Autodesk Fusion 360 part; units mm, degrees
(part 2 of 3)
sketch "plate_cut" plane through (0, 0, 0) normal (0, 1, 0) x (1, 0, 0)
  arc A0 (26.05, -31.55) -> (25.05, -32.55) centre (25.05, -31.55) cw
  arc A1 (13.05, -32.55) -> (12.05, -31.55) centre (13.05, -31.55) cw
  line L0 (1.286, -37.6) -> (13.286, -37.6)
  line L1 (14.286, -38.6) -> (14.286, -50.6)
  line L2 (23.2714, -39.7827) -> (20.1656, -51.3738)
  arc A2 (14.286, -50.6) -> (13.286, -51.6) centre (13.286, -50.6) cw
  arc A3 (36.7944, -43.4062) -> (36.0873, -42.1814) centre (35.8285, -43.1474) ccw
  arc A4 (32.4638, -55.7044) -> (33.6886, -54.9973) centre (32.7226, -54.7385) ccw
  arc A5 (13.286, -37.6) -> (14.286, -38.6) centre (13.286, -38.6) cw
  arc A6 (24.4962, -39.0756) -> (23.2714, -39.7827) centre (24.2374, -40.0415) ccw
  line L3 (59.2962, -48.3878) -> (48.9038, -42.3878)
  line L4 (25.05, -32.55) -> (13.05, -32.55)
  arc A7 (32.1, -35.05) -> (31.1, -34.05) centre (32.1, -34.05) cw
  arc A8 (20.1656, -51.3738) -> (20.8727, -52.5986) centre (21.1315, -51.6326) ccw
  line L5 (20.8727, -52.5986) -> (32.4638, -55.7044)
  line L6 (13.286, -51.6) -> (1.286, -51.6)
  arc A9 (-7, 6) -> (-6, 7) centre (-6, 6) cw
  line L7 (-13.05, 6.05) -> (-25.05, 6.05)
  line L8 (-7, -6) -> (-7, 6)
  line L9 (47.5378, -42.7538) -> (41.5378, -53.1462)
  arc A10 (26.05, -12.5) -> (25.05, -13.5) centre (25.05, -12.5) cw
  arc A11 (6, 7) -> (7, 6) centre (6, 6) cw
  line L10 (-12.05, -19.06) -> (-12.05, -31.06)
  arc A12 (12.05, -19.55) -> (13.05, -18.55) centre (13.05, -19.55) cw
  line L11 (45.1, -22.05) -> (45.1, -34.05)
  arc A13 (-12.05, 7.05) -> (-13.05, 6.05) centre (-13.05, 7.05) cw
  arc A14 (-6, -26.05) -> (-7, -25.05) centre (-6, -25.05) cw
  arc A15 (1.286, -51.6) -> (0.286, -50.6) centre (1.286, -50.6) cw
  arc A16 (-13.05, -18.06) -> (-12.05, -19.06) centre (-13.05, -19.06) cw
  arc A17 (-13.05, 1) -> (-12.05, 0) centre (-13.05, 0) cw
  line L12 (12.05, -12.5) -> (12.05, -0.5)
  line L13 (6, -26.05) -> (-6, -26.05)
  line L14 (-25.05, 1) -> (-13.05, 1)
  arc A18 (-6, -7) -> (-7, -6) centre (-6, -6) cw
  arc A19 (12.05, -0.5) -> (13.05, 0.5) centre (13.05, -0.5) cw
  line L15 (7, -13.05) -> (7, -25.05)
  line L16 (-45.1, -43.05) -> (-45.1, -31.05)
  line L17 (-32.1, -25) -> (-44.1, -25)
  line L18 (53.6622, -60.1462) -> (59.6622, -49.7538)
  arc A20 (41.5378, -53.1462) -> (41.9038, -54.5122) centre (42.4038, -53.6462) ccw
  line L19 (13.05, 0.5) -> (25.05, 0.5)
  arc A21 (-26.05, -19.06) -> (-25.05, -18.06) centre (-25.05, -19.06) cw
  line L20 (44.1, 3.05) -> (32.1, 3.05)
  line L21 (-44.1, -30.05) -> (-32.1, -30.05)
  arc A22 (-45.1, -12) -> (-44.1, -11) centre (-44.1, -12) cw
  arc A23 (13.05, 5.55) -> (12.05, 6.55) centre (13.05, 6.55) cw
  arc A24 (25.05, -18.55) -> (26.05, -19.55) centre (25.05, -19.55) cw
  line L22 (-6, 7) -> (6, 7)
  arc A25 (-32.1, -30.05) -> (-31.1, -31.05) centre (-32.1, -31.05) cw
  line L23 (31.1, 4.05) -> (31.1, 16.05)
  line L24 (-31.1, -31.05) -> (-31.1, -43.05)
  line L25 (32.1, 17.05) -> (44.1, 17.05)
  line L26 (12.05, 6.55) -> (12.05, 18.55)
  line L27 (26.05, 18.55) -> (26.05, 6.55)
  line L28 (-44.1, -11) -> (-32.1, -11)
  line L29 (25.05, 5.55) -> (13.05, 5.55)
  arc A26 (45.1, 4.05) -> (44.1, 3.05) centre (44.1, 4.05) cw
  line L30 (-32.1, -44.05) -> (-44.1, -44.05)
  arc A27 (32.1, 3.05) -> (31.1, 4.05) centre (32.1, 4.05) cw
  line L31 (13.05, 19.55) -> (25.05, 19.55)
  line L32 (45.1, 16.05) -> (45.1, 4.05)
  line L33 (41.9038, -54.5122) -> (52.2962, -60.5122)
  line L34 (-12.05, 0) -> (-12.05, -12)
  line L35 (-26.05, -12) -> (-26.05, 0)
  arc A28 (59.6622, -49.7538) -> (59.2962, -48.3878) centre (58.7962, -49.2538) ccw
  arc A29 (48.9038, -42.3878) -> (47.5378, -42.7538) centre (48.4038, -43.2538) ccw
  line L36 (44.1, -35.05) -> (32.1, -35.05)
  line L37 (36.0873, -42.1814) -> (24.4962, -39.0756)
  line L38 (33.6886, -54.9973) -> (36.7944, -43.4062)
  line L39 (-7, -25.05) -> (-7, -13.05)
  arc A30 (25.05, 0.5) -> (26.05, -0.5) centre (25.05, -0.5) cw
  arc A31 (44.1, 17.05) -> (45.1, 16.05) centre (44.1, 16.05) cw
  arc A32 (45.1, -34.05) -> (44.1, -35.05) centre (44.1, -34.05) cw
  arc A33 (0.286, -38.6) -> (1.286, -37.6) centre (1.286, -38.6) cw
  arc A34 (7, -6) -> (6, -7) centre (6, -6) cw
  line L40 (-25.05, 20.05) -> (-13.05, 20.05)
  line L41 (6, -7) -> (-6, -7)
  arc A35 (13.05, -13.5) -> (12.05, -12.5) centre (13.05, -12.5) cw
  arc A36 (7, -25.05) -> (6, -26.05) centre (6, -25.05) cw
  line L42 (13.05, -18.55) -> (25.05, -18.55)
  line L43 (7, 6) -> (7, -6)
  line L44 (25.05, -13.5) -> (13.05, -13.5)
  arc A37 (-7, -13.05) -> (-6, -12.05) centre (-6, -13.05) cw
  line L45 (26.05, -0.5) -> (26.05, -12.5)
  arc A38 (6, -12.05) -> (7, -13.05) centre (6, -13.05) cw
  arc A39 (-12.05, -12) -> (-13.05, -13) centre (-13.05, -12) cw
  line L46 (0.286, -50.6) -> (0.286, -38.6)
  arc A40 (-12.05, -31.06) -> (-13.05, -32.06) centre (-13.05, -31.06) cw
  line L47 (26.05, -19.55) -> (26.05, -31.55)
  line L48 (-6, -12.05) -> (6, -12.05)
  line L49 (-6, 26.05) -> (6, 26.05)
  arc A41 (32.1, -16) -> (31.1, -15) centre (32.1, -15) cw
  line L50 (32.1, -21.05) -> (44.1, -21.05)
  line L51 (7, 25.05) -> (7, 13.05)
  arc A42 (44.1, -21.05) -> (45.1, -22.05) centre (44.1, -22.05) cw
  arc A43 (-26.05, 19.05) -> (-25.05, 20.05) centre (-25.05, 19.05) cw
  arc A44 (7, 13.05) -> (6, 12.05) centre (6, 13.05) cw
  arc A45 (31.1, -22.05) -> (32.1, -21.05) centre (32.1, -22.05) cw
  arc A46 (-44.1, 8.05) -> (-45.1, 7.05) centre (-44.1, 7.05) ccw
  line L52 (44.1, -16) -> (32.1, -16)
  arc A47 (-25.05, 6.05) -> (-26.05, 7.05) centre (-25.05, 7.05) cw
  arc A48 (-13.05, 20.05) -> (-12.05, 19.05) centre (-13.05, 19.05) cw
  line L53 (32.1, -2) -> (44.1, -2)
  arc A49 (31.1, -3) -> (32.1, -2) centre (32.1, -3) cw
  line L54 (-26.05, 7.05) -> (-26.05, 19.05)
  line L55 (31.1, -15) -> (31.1, -3)
  arc A50 (45.1, -15) -> (44.1, -16) centre (44.1, -15) cw
  arc A51 (6, 26.05) -> (7, 25.05) centre (6, 25.05) cw
  line L56 (-31.1, -4.95) -> (-31.1, 7.05)
  line L57 (-31.1, -12) -> (-31.1, -24)
  arc A52 (44.1, -2) -> (45.1, -3) centre (44.1, -3) cw
  line L58 (-44.1, -5.95) -> (-32.1, -5.95)
  arc A53 (-32.1, -11) -> (-31.1, -12) centre (-32.1, -12) cw
  arc A54 (-32.1, -5.95) -> (-31.1, -4.95) centre (-32.1, -4.95) ccw
  line L59 (45.1, -3) -> (45.1, -15)
  line L60 (-7, 13.05) -> (-7, 25.05)
  arc A55 (-7, 25.05) -> (-6, 26.05) centre (-6, 25.05) cw
  arc A56 (-44.1, -25) -> (-45.1, -24) centre (-44.1, -24) cw
  line L61 (-26.05, -31.06) -> (-26.05, -19.06)
  arc A57 (-6, 12.05) -> (-7, 13.05) centre (-6, 13.05) cw
  line L62 (-45.1, 7.05) -> (-45.1, -4.95)
  arc A58 (-25.05, -32.06) -> (-26.05, -31.06) centre (-25.05, -31.06) cw
  line L63 (-32.1, 8.05) -> (-44.1, 8.05)
  line L64 (6, 12.05) -> (-6, 12.05)
  arc A59 (-31.1, -43.05) -> (-32.1, -44.05) centre (-32.1, -43.05) cw
  arc A60 (-26.05, 0) -> (-25.05, 1) centre (-25.05, 0) cw
  arc A61 (-31.1, -24) -> (-32.1, -25) centre (-32.1, -24) cw
  line L65 (-12.05, 19.05) -> (-12.05, 7.05)
  arc A62 (25.05, 19.55) -> (26.05, 18.55) centre (25.05, 18.55) cw
  arc A63 (12.05, 18.55) -> (13.05, 19.55) centre (13.05, 18.55) cw
  line L66 (-45.1, -24) -> (-45.1, -12)
  arc A64 (-31.1, 7.05) -> (-32.1, 8.05) centre (-32.1, 7.05) ccw
  line L67 (-25.05, -18.06) -> (-13.05, -18.06)
  arc A65 (31.1, 16.05) -> (32.1, 17.05) centre (32.1, 16.05) cw
  arc A66 (-45.1, -31.05) -> (-44.1, -30.05) centre (-44.1, -31.05) cw
  line L68 (31.1, -34.05) -> (31.1, -22.05)
  arc A67 (-45.1, -4.95) -> (-44.1, -5.95) centre (-44.1, -4.95) ccw
  line L69 (-13.05, -32.06) -> (-25.05, -32.06)
  arc A68 (26.05, 6.55) -> (25.05, 5.55) centre (25.05, 6.55) cw
  arc A69 (-25.05, -13) -> (-26.05, -12) centre (-25.05, -12) cw
  line L70 (-13.05, -13) -> (-25.05, -13)
  line L71 (12.05, -31.55) -> (12.05, -19.55)
  arc A70 (-44.1, -44.05) -> (-45.1, -43.05) centre (-44.1, -43.05) cw
  arc A71 (52.2962, -60.5122) -> (53.6622, -60.1462) centre (52.7962, -59.6462) ccw
  arc A72 (-55.7487, 17.9209) -> (-60.125, 9.652) centre (-50.125, 9.652) ccw
  line L72 (-55.7487, 17.9209) -> (-24.2468, 39.3454)
  arc A73 (-18.6222, 41.0765) -> (-24.2468, 39.3454) centre (-18.6231, 31.0765) ccw
  line L73 (-18.6222, 41.0765) -> (18.4843, 41.0734)
  arc A74 (20.6567, 40.8344) -> (18.4843, 41.0734) centre (18.4835, 31.0734) ccw
  arc A75 (81.043, 19.3715) -> (73.2162, 29.1325) centre (71.043, 19.3715) ccw
  arc A76 (79.7028, -45.0985) -> (81.043, -40.0977) centre (71.043, -40.0977) ccw
  line L74 (79.7028, -45.0985) -> (61.8222, -76.0618)
  arc A77 (53.2987, -81.06) -> (61.8222, -76.0618) centre (53.1625, -71.0609) ccw
  line L75 (53.2987, -81.06) -> (29.1948, -81.3885)
  arc A78 (24.8527, -80.462) -> (29.1948, -81.3885) centre (29.0585, -71.3894) ccw
  line L76 (24.8527, -80.462) -> (-19.2813, -60.0025)
  arc A79 (-19.2813, -60.0025) -> (-23.4871, -59.075) centre (-23.4871, -69.075) ccw
  line L77 (-50.125, -59.075) -> (-23.4871, -59.075)
  arc A80 (-60.125, -49.075) -> (-50.125, -59.075) centre (-50.125, -49.075) ccw
  line L78 (-60.125, -49.075) -> (-60.125, 9.652)
  line L79 (20.6567, 40.8344) -> (46.8423, 35.0044)
  line L80 (81.043, 19.3715) -> (81.043, -25.8559)
  arc A81 (47.625, 34.0283) -> (46.8423, 35.0044) centre (46.625, 34.0283) ccw
  line L81 (47.625, 34.0283) -> (47.625, -32.5721)
  line L82 (69.2205, -25.8646) -> (69.0694, 28.8059)
  arc A82 (70.2867, 29.7847) -> (69.0694, 28.8059) centre (70.0694, 28.8086) ccw
  arc A83 (47.625, -32.5721) -> (48.1249, -33.4381) centre (48.625, -32.5721) ccw
  line L83 (48.1249, -33.4381) -> (57.1204, -38.6328)
  arc A84 (57.1204, -38.6328) -> (57.6205, -38.7668) centre (57.6205, -37.7668) ccw
  line L84 (70.2211, -26.8618) -> (80.0436, -26.8559)
  arc A85 (69.2205, -25.8646) -> (70.2211, -26.8618) centre (70.2205, -25.8618) ccw
  arc A86 (80.0436, -26.8559) -> (81.043, -25.8559) centre (80.043, -25.8559) ccw
  line L85 (57.6205, -38.7668) -> (80.043, -38.7668)
  arc A87 (81.043, -39.7668) -> (80.043, -38.7668) centre (80.043, -39.7668) ccw
  line L86 (81.043, -39.7668) -> (81.043, -40.0977)
  circle A88 centre (71.1231, -41.9588) radius 1.7
  circle A89 centre (53.7342, -72.0705) radius 1.7
  circle A90 centre (28.4977, -72.2317) radius 1.7
  circle A91 centre (-18.212, -50.5781) radius 1.7
  circle A92 centre (-51.125, -50.075) radius 1.7
  circle A93 centre (-51.125, 10.1813) radius 1.7
  circle A94 centre (-18.9309, 32.0765) radius 1.7
  circle A95 centre (18.5935, 32.0734) radius 1.7
  circle A96 centre (43.1794, 26.5995) radius 1.7
  circle A97 centre (72.0934, 20.1391) radius 1.7
  circle A98 centre (72.2122, -22.8606) radius 1.7
  line L87 (70.2867, 29.7847) -> (73.2162, 29.1325)
sketch "curve_measure" plane through (0, 0, 0) normal (0, 0, 1) x (1, 0, 0)
  line L0 (75, 8.5) -> (75, -1.5)
  line L1 (75, -1.5) -> (81, -1.5)
  line L2 (81, -1.5) -> (81, 8.5)
  line L3 (81, 8.5) -> (75, 8.5)
  line L4 (73.5, 6) -> (82.5, 6) construction
  line L5 (82, 3) -> (73.5, 3) construction
  line L6 (79.7028, 0) -> (61.8222, 0) construction
  line L7 (80.5, -0.5199) -> (80.5, 9.6972) construction
  line L8 (79.25, 9.8527) -> (79.25, -0.7376) construction
  dimension "d106" = 3
  dimension "d107" = 2.5
  dimension "d108" = 0.5
  dimension "d109" = 1.75
  dimension "d110" = 6
  constraint vertical L0
  constraint perpendicular L0 L1
  constraint perpendicular L1 L2
  constraint perpendicular L0 L3
  constraint perpendicular L2 L4
  constraint perpendicular L0 L5
  constraint perpendicular L3 L7
  constraint vertical L8
  measures "d106" distance of L5 L6
  measures "d107" distance of L3 L4
  measures "d108" distance of L2 L7
  measures "d109" distance of L2 L8
  measures "d110" distance of L0 L2
extrude "Extrude2" add sketch "plate_cut" against normal blind 1.6 makes body 1 at (2.2858, 0, 64.0215) makes body 2 at (75.5302, 0, -5.55)
sketch "key_outline" plane through (0, 0, 0) normal (0, 1, 0) x (1, 0, 0)
  line L0 (-47.625, 10.575) -> (-28.575, 10.575)
  line L1 (-28.575, 10.575) -> (-28.575, 22.575)
  line L2 (-28.575, 22.575) -> (-9.525, 22.575)
  line L3 (-9.525, 22.575) -> (-9.525, 28.575)
  line L4 (-9.525, 28.575) -> (9.525, 28.575)
  line L5 (9.525, 28.575) -> (9.525, 22.075)
  line L6 (9.525, 22.075) -> (28.575, 22.075)
  line L7 (28.575, 22.075) -> (28.575, 19.575)
  line L8 (28.575, 19.575) -> (47.625, 19.575)
  line L9 (47.625, 19.575) -> (47.625, -33.2267)
  line L10 (47.625, -33.2267) -> (65.9971, -43.8338)
  line L11 (65.9971, -43.8338) -> (51.7096, -68.5805)
  line L12 (51.7096, -68.5805) -> (35.2118, -59.0555)
  line L13 (35.2118, -59.0555) -> (16.8109, -54.125)
  line L14 (16.8109, -54.125) -> (-2.2391, -54.125)
  line L15 (-2.2391, -54.125) -> (-2.2391, -35.075)
  line L16 (-9.525, -34.575) -> (-28.575, -34.575)
  line L17 (-28.575, -34.575) -> (-28.575, -46.575)
  line L18 (-28.575, -46.575) -> (-47.625, -46.575)
  line L19 (-47.625, -46.575) -> (-47.625, 10.575)
  line L20 (-2.2391, -35.075) -> (-2.2391, -34.575)
  line L21 (-9.525, -34.575) -> (-2.2391, -34.575)
  line L22 (-9.525, -35.575) -> (-3.2391, -35.575)
  line L23 (-9.525, -35.575) -> (-27.575, -35.575)
  line L24 (-27.575, -35.575) -> (-27.575, -47.575)
  line L25 (-27.575, -47.575) -> (-48.625, -47.575)
  line L26 (-48.625, -47.575) -> (-48.625, 11.575)
  line L27 (-48.625, 11.575) -> (-29.575, 11.575)
  line L28 (-29.575, 11.575) -> (-29.575, 23.575)
  line L29 (-29.575, 23.575) -> (-10.525, 23.575)
  line L30 (-10.525, 23.575) -> (-10.525, 29.575)
  line L31 (-10.525, 29.575) -> (10.525, 29.575)
  line L32 (10.525, 29.575) -> (10.525, 23.075)
  line L33 (10.525, 23.075) -> (29.575, 23.075)
  line L34 (29.575, 23.075) -> (29.575, 20.575)
  line L35 (29.575, 20.575) -> (48.625, 20.575)
  line L36 (48.625, 20.575) -> (48.625, -32.6494)
  line L37 (48.625, -32.6494) -> (67.3631, -43.4678)
  line L38 (67.3631, -43.4678) -> (52.0756, -69.9465)
  line L39 (52.0756, -69.9465) -> (34.8258, -59.9874)
  line L40 (34.8258, -59.9874) -> (16.6792, -55.125)
  line L41 (16.6792, -55.125) -> (-3.2391, -55.125)
  line L42 (-3.2391, -55.125) -> (-3.2391, -35.575)
  point P0 (-47.625, 10.575)
  point P1 (-28.575, 10.575)
  point P2 (-28.575, 22.575)
  point P3 (-9.525, 22.575)
  point P4 (-9.525, 28.575)
  point P5 (9.525, 28.575)
  point P6 (9.525, 22.075)
  point P7 (28.575, 22.075)
  point P8 (28.575, 19.575)
  point P9 (47.625, 19.575)
  point P10 (47.625, -33.2267)
  point P11 (65.9971, -43.8338)
  point P12 (51.7096, -68.5805)
  point P13 (35.2118, -59.0555)
  point P14 (16.8109, -54.125)
  point P15 (-2.2391, -54.125)
  point P16 (-2.2391, -35.075)
  point P17 (-9.525, -34.575)
  point P18 (-28.575, -34.575)
  point P19 (-28.575, -46.575)
  point P20 (-47.625, -46.575)
  dimension "d128" = 1
  constraint coincident P0 L0.start
  constraint coincident P1 L0.end
  constraint coincident P2 L1.end
  constraint coincident P3 L2.end
  constraint coincident P4 L3.end
  constraint coincident P5 L4.end
  constraint coincident P6 L5.end
  constraint coincident P7 L6.end
  constraint coincident P8 L7.end
  constraint coincident P9 L8.end
  constraint coincident P10 L9.end
  constraint coincident P11 L10.end
  constraint coincident P12 L11.end
  constraint coincident P13 L12.end
  constraint coincident P14 L13.end
  constraint coincident P15 L14.end
  constraint coincident P16 L15.end
  constraint coincident P17 L16.start
  constraint coincident P18 L16.end
  constraint coincident P19 L17.end
  constraint coincident P20 L18.end
sketch "top_c" plane through (0, 0, 0) normal (0, 1, 0) x (1, 0, 0)
  line L0 (-48.625, 11.575) -> (-29.575, 11.575)
  line L1 (-48.625, -47.575) -> (-48.625, 11.575)
  line L2 (-29.575, 11.575) -> (-29.575, 23.575)
  line L3 (-29.575, 23.575) -> (-10.525, 23.575)
  line L4 (-10.525, 29.575) -> (10.525, 29.575)
  line L5 (-10.525, 23.575) -> (-10.525, 29.575)
  line L6 (10.525, 29.575) -> (10.525, 23.075)
  line L7 (10.525, 23.075) -> (29.575, 23.075)
  line L8 (29.575, 23.075) -> (29.575, 20.575)
  line L9 (29.575, 20.575) -> (48.625, 20.575)
  line L10 (48.625, 20.575) -> (48.625, -32.6494)
  line L11 (48.625, -32.6494) -> (67.3631, -43.4678)
  line L12 (67.3631, -43.4678) -> (52.0756, -69.9465)
  line L13 (52.0756, -69.9465) -> (34.8258, -59.9874)
  line L14 (34.8258, -59.9874) -> (16.6792, -55.125)
  line L15 (16.6792, -55.125) -> (-3.2391, -55.125)
  line L16 (-3.2391, -55.125) -> (-3.2391, -35.575)
  line L17 (-9.525, -35.575) -> (-3.2391, -35.575)
  line L18 (-9.525, -35.575) -> (-27.575, -35.575)
  line L19 (-27.575, -35.575) -> (-27.575, -47.575)
  line L20 (-27.575, -47.575) -> (-48.625, -47.575)
  line L21 (-18.6227, 35.5765) -> (18.4839, 35.5734)
  arc A0 (19.4614, 35.4658) -> (18.4839, 35.5734) centre (18.4835, 31.0734) ccw
  line L22 (19.4614, 35.4658) -> (45.6471, 29.6358)
  circle A1 centre (18.5935, 32.0734) radius 1.1
  circle A2 centre (43.1794, 26.5995) radius 1.1
  circle A3 centre (-18.9309, 32.0765) radius 1.1
  arc A4 (-18.6227, 35.5765) -> (-21.1537, 34.7975) centre (-18.6231, 31.0765) ccw
  line L23 (-52.6557, 13.373) -> (-21.1537, 34.7975)
  line L24 (45.6471, 29.6358) -> (70.2803, 24.3774)
  line L25 (72.0209, 23.7639) -> (70.2803, 24.3774)
  arc A5 (75.543, 19.3715) -> (72.0209, 23.7639) centre (71.043, 19.3715) ccw
  circle A6 centre (72.0934, 20.1391) radius 1.1
  line L26 (75.543, 19.3715) -> (75.543, -25.8607)
  line L27 (75.543, -25.8607) -> (75.543, -40.0977)
  arc A7 (74.9399, -42.3481) -> (75.543, -40.0977) centre (71.043, -40.0977) ccw
  line L28 (74.9399, -42.3481) -> (57.0594, -73.3113)
  arc A8 (53.2238, -75.5605) -> (57.0594, -73.3113) centre (53.1625, -71.0609) ccw
  circle A9 centre (53.7342, -72.0705) radius 1.1
  circle A10 centre (71.1231, -41.9588) radius 1.1
  circle A11 centre (28.4977, -72.2317) radius 1.1
  arc A12 (27.1659, -75.4721) -> (29.1198, -75.889) centre (29.0585, -71.3894) ccw
  line L29 (27.1659, -75.4721) -> (-16.9681, -55.0126)
  arc A13 (-16.9681, -55.0126) -> (-23.4871, -53.575) centre (-23.4871, -69.075) ccw
  line L30 (-50.125, -53.575) -> (-23.4871, -53.575)
  arc A14 (-54.625, -49.075) -> (-50.125, -53.575) centre (-50.125, -49.075) ccw
  line L31 (-54.625, -49.075) -> (-54.625, 9.652)
  circle A15 centre (-51.125, -50.075) radius 1.1
  circle A16 centre (-18.212, -50.5781) radius 1.1
  arc A17 (-52.6557, 13.373) -> (-54.625, 9.652) centre (-50.125, 9.652) ccw
  circle A18 centre (-51.125, 10.1813) radius 1.1
  line L32 (53.2238, -75.5605) -> (29.1198, -75.889)
  circle A19 centre (72.2122, -22.8606) radius 1.1
sketch "top_b" plane through (0, 0, 0) normal (0, 1, 0) x (1, 0, 0)
  line L0 (-48.625, -47.575) -> (-48.625, 11.575)
  line L1 (-48.625, 11.575) -> (-29.575, 11.575)
  line L2 (-29.575, 11.575) -> (-29.575, 23.575)
  line L3 (-29.575, 23.575) -> (-10.525, 23.575)
  line L4 (-10.525, 29.575) -> (10.525, 29.575)
  line L5 (-10.525, 23.575) -> (-10.525, 29.575)
  line L6 (10.525, 29.575) -> (10.525, 23.075)
  line L7 (10.525, 23.075) -> (29.575, 23.075)
  line L8 (29.575, 23.075) -> (29.575, 20.575)
  line L9 (67.3631, -43.4678) -> (52.0756, -69.9465)
  line L10 (52.0756, -69.9465) -> (34.8258, -59.9874)
  line L11 (34.8258, -59.9874) -> (16.6792, -55.125)
  line L12 (16.6792, -55.125) -> (-3.2391, -55.125)
  line L13 (-3.2391, -55.125) -> (-3.2391, -35.575)
  line L14 (-9.525, -35.575) -> (-3.2391, -35.575)
  line L15 (-9.525, -35.575) -> (-27.575, -35.575)
  line L16 (-27.575, -35.575) -> (-27.575, -47.575)
  line L17 (-27.575, -47.575) -> (-48.625, -47.575)
  line L18 (-54.7645, 16.4738) -> (-23.2626, 37.8983)
  arc A0 (-18.6224, 39.3265) -> (-23.2626, 37.8983) centre (-18.6231, 31.0765) ccw
  line L19 (-18.6224, 39.3265) -> (18.4842, 39.3234)
  circle A1 centre (-18.9309, 32.0765) radius 1.7
  circle A2 centre (18.5935, 32.0734) radius 1.7
  circle A3 centre (-51.125, 10.1813) radius 1.7
  arc A4 (-54.7645, 16.4738) -> (-58.375, 9.652) centre (-50.125, 9.652) ccw
  line L20 (-58.375, -49.075) -> (-58.375, 9.652)
  arc A5 (-58.375, -49.075) -> (-50.125, -57.325) centre (-50.125, -49.075) ccw
  circle A6 centre (-51.125, -50.075) radius 1.7
  circle A7 centre (-18.212, -50.5781) radius 1.7
  line L21 (-50.125, -57.325) -> (-23.4871, -57.325)
  arc A8 (-18.5453, -58.4148) -> (-23.4871, -57.325) centre (-23.4871, -69.075) ccw
  line L22 (25.5887, -78.8743) -> (-18.5453, -58.4148)
  arc A9 (25.5887, -78.8743) -> (29.1709, -79.6387) centre (29.0585, -71.3894) ccw
  line L23 (53.2749, -79.3102) -> (29.1709, -79.6387)
  arc A10 (53.2749, -79.3102) -> (60.3068, -75.1866) centre (53.1625, -71.0609) ccw
  line L24 (78.1873, -44.2234) -> (60.3068, -75.1866)
  arc A11 (78.1873, -44.2234) -> (79.293, -40.0977) centre (71.043, -40.0977) ccw
  circle A12 centre (71.1231, -41.9588) radius 1.7
  circle A13 centre (53.7342, -72.0705) radius 1.7
  circle A14 centre (72.1849, -22.8607) radius 1.7
  arc A15 (78.293, -26.8607) -> (79.293, -25.8607) centre (78.293, -25.8607) ccw
  line L25 (79.293, 19.3715) -> (79.293, -25.8607)
  arc A16 (69.1916, -25.8629) -> (70.1916, -26.8607) centre (70.1916, -25.8607) ccw
  arc A17 (79.293, 19.3715) -> (72.8359, 27.4243) centre (71.043, 19.3715) ccw
  line L26 (72.8359, 27.4243) -> (70.2865, 28.1461)
  arc A18 (70.2865, 28.1461) -> (69.0691, 27.1678) centre (70.0691, 27.17) ccw
  circle A19 centre (72.1849, 20.1393) radius 1.7
  circle A20 centre (43.1794, 26.5995) radius 1.7
  line L27 (20.2764, 39.1262) -> (46.462, 33.2962)
  arc A21 (20.2764, 39.1262) -> (18.4842, 39.3234) centre (18.4835, 31.0734) ccw
  line L28 (59.2208, -38.7668) -> (78.293, -38.7668)
  line L29 (47.625, 32.2354) -> (47.625, 20.575)
  line L30 (70.1916, -26.8607) -> (78.293, -26.8607)
  line L31 (69.1916, -25.8629) -> (69.0729, 27.2561)
  line L32 (59.2208, -38.7668) -> (67.3631, -43.4678)
  line L33 (79.293, -40.0977) -> (79.293, -39.7668)
  arc A22 (79.293, -39.7668) -> (78.293, -38.7668) centre (78.293, -39.7668) ccw
  line L34 (46.462, 33.2962) -> (46.8423, 33.2115)
  arc A23 (47.625, 32.2354) -> (46.8423, 33.2115) centre (46.625, 32.2354) ccw
  line L35 (29.575, 20.575) -> (47.625, 20.575)
  circle A24 centre (28.4977, -72.2317) radius 1.7
  dimension "d132" = 1
  dimension "d133" = 1
  constraint coincident A18 L31.end
  constraint coincident L9.start L32.end
  constraint perpendicular L9 L32
  constraint tangent A11 L33
  constraint vertical L33
  constraint tangent L28 A22
  constraint tangent L33 A22
  constraint parallel L27 L34
  constraint tangent L34 A23
  constraint tangent L29 A23
  constraint coincident L8.end L35.start
  constraint perpendicular L8 L35
  measures "d132" radius of A22
  measures "d133" radius of A23
sketch "top_a" plane through (0, 0, 0) normal (0, 1, 0) x (1, 0, 0)
  line L0 (29.575, 23.075) -> (29.575, 20.575)
  line L1 (10.525, 23.075) -> (29.575, 23.075)
  line L2 (10.525, 29.575) -> (10.525, 23.075)
  line L3 (-10.525, 29.575) -> (10.525, 29.575)
  line L4 (-10.525, 23.575) -> (-10.525, 29.575)
  line L5 (-29.575, 23.575) -> (-10.525, 23.575)
  line L6 (-29.575, 11.575) -> (-29.575, 23.575)
  line L7 (-48.625, 11.575) -> (-29.575, 11.575)
  line L8 (-48.625, -47.575) -> (-48.625, 11.575)
  line L9 (-27.575, -47.575) -> (-48.625, -47.575)
  line L10 (-27.575, -35.575) -> (-27.575, -47.575)
  line L11 (-9.525, -35.575) -> (-27.575, -35.575)
  line L12 (-9.525, -35.575) -> (-3.2391, -35.575)
  line L13 (-3.2391, -55.125) -> (-3.2391, -35.575)
  line L14 (16.6792, -55.125) -> (-3.2391, -55.125)
  line L15 (34.8258, -59.9874) -> (16.6792, -55.125)
  line L16 (52.0756, -69.9465) -> (34.8258, -59.9874)
  line L17 (67.3631, -43.4678) -> (52.0756, -69.9465)
  line L18 (20.548, 40.3463) -> (46.7337, 34.5163)
  arc A0 (20.548, 40.3463) -> (18.4843, 40.5734) centre (18.4835, 31.0734) ccw
  line L19 (-18.6223, 40.5765) -> (18.4843, 40.5734)
  arc A1 (-18.6223, 40.5765) -> (-23.9656, 38.9319) centre (-18.6231, 31.0765) ccw
  line L20 (-55.4675, 17.5074) -> (-23.9656, 38.9319)
  arc A2 (-55.4675, 17.5074) -> (-59.625, 9.652) centre (-50.125, 9.652) ccw
  line L21 (-59.625, -49.075) -> (-59.625, 9.652)
  arc A3 (-59.625, -49.075) -> (-50.125, -58.575) centre (-50.125, -49.075) ccw
  line L22 (-50.125, -58.575) -> (-23.4871, -58.575)
  arc A4 (-19.071, -59.5488) -> (-23.4871, -58.575) centre (-23.4871, -69.075) ccw
  line L23 (25.063, -80.0083) -> (-19.071, -59.5488)
  arc A5 (25.063, -80.0083) -> (29.1879, -80.8885) centre (29.0585, -71.3894) ccw
  line L24 (53.2919, -80.5601) -> (29.1879, -80.8885)
  arc A6 (53.2919, -80.5601) -> (61.3893, -75.8117) centre (53.1625, -71.0609) ccw
  line L25 (79.2698, -44.8485) -> (61.3893, -75.8117)
  arc A7 (79.2698, -44.8485) -> (80.5358, -39.7279) centre (71.043, -40.0977) ccw
  line L26 (69.1916, -25.8629) -> (69.0702, 28.465)
  line L27 (73.1075, 28.6444) -> (70.2865, 29.3961)
  arc A8 (80.543, 19.3715) -> (73.1075, 28.6444) centre (71.043, 19.3715) ccw
  line L28 (80.543, 19.3715) -> (80.543, -25.8607)
  arc A9 (79.543, -26.8607) -> (80.543, -25.8607) centre (79.543, -25.8607) ccw
  line L29 (70.1916, -26.8607) -> (79.543, -26.8607)
  arc A10 (69.1916, -25.8629) -> (70.1916, -26.8607) centre (70.1916, -25.8607) ccw
  circle A11 centre (72.1849, -22.8607) radius 1.7
  circle A12 centre (72.1849, 20.1393) radius 1.7
  circle A13 centre (43.1794, 26.5995) radius 1.7
  circle A14 centre (18.5935, 32.0734) radius 1.7
  circle A15 centre (-18.9309, 32.0765) radius 1.7
  circle A16 centre (-51.125, 10.1813) radius 1.7
  circle A17 centre (-51.125, -50.075) radius 1.7
  circle A18 centre (-18.212, -50.5781) radius 1.7
  circle A19 centre (28.4977, -72.2317) radius 1.7
  circle A20 centre (53.7342, -72.0705) radius 1.7
  circle A21 centre (71.1231, -41.9588) radius 1.7
  line L30 (59.2208, -38.7668) -> (79.5366, -38.7668)
  arc A22 (80.5358, -39.7279) -> (79.5366, -38.7668) centre (79.5366, -39.7668) ccw
  line L31 (67.3631, -43.4678) -> (59.2208, -38.7668)
  line L32 (47.625, 20.575) -> (47.625, 33.516)
  line L33 (46.7337, 34.5163) -> (46.8423, 34.4921)
  arc A23 (47.625, 33.516) -> (46.8423, 34.4921) centre (46.625, 33.516) ccw
  line L34 (29.575, 20.575) -> (47.625, 20.575)
  line L35 (70.2865, 29.3961) -> (70.3273, 29.3852)
  line L36 (69.0702, 28.465) -> (69.0699, 28.4264)
  arc A24 (70.3273, 29.3852) -> (69.0699, 28.4264) centre (70.0698, 28.4189) ccw
  dimension "d134" = 1
  dimension "d135" = 1
  dimension "d138" = 1
  constraint tangent L30 A22
  constraint tangent A7 A22
  constraint coincident L17.start L31.start
  constraint perpendicular L17 L31
  constraint parallel L18 L33
  constraint tangent L33 A23
  constraint tangent L32 A23
  constraint coincident L0.end L34.start
  constraint perpendicular L32 L34
  constraint parallel L27 L35
  constraint tangent L36 A24
  constraint tangent L35 A24
  measures "d134" radius of A22
  measures "d135" radius of A23
  measures "d138" radius of A24
sketch "bottom_a" plane through (0, 0, 0) normal (0, 1, 0) x (1, 0, 0)
  line L0 (45.6471, 29.6358) -> (69.7865, 24.3961)
  circle A0 centre (72.1849, -22.8607) radius 1.1
  circle A1 centre (72.1849, 20.1393) radius 1.1
  arc A2 (27.1659, -75.4721) -> (29.1198, -75.889) centre (29.0585, -71.3894) ccw
  circle A3 centre (28.4977, -72.2317) radius 1.1
  line L1 (53.2238, -75.5605) -> (29.1198, -75.889)
  arc A4 (75.543, 19.3715) -> (72.0209, 23.7639) centre (71.043, 19.3715) ccw
  circle A5 centre (43.1794, 26.5995) radius 1.1
  line L2 (27.1659, -75.4721) -> (-16.9681, -55.0126)
  line L3 (75.543, 19.3715) -> (75.543, -25.8607)
  line L4 (72.0209, 23.7639) -> (69.7865, 24.3961)
  line L5 (-54.625, -49.075) -> (-54.625, 9.652)
  circle A6 centre (71.1231, -41.9588) radius 1.1
  arc A7 (53.2238, -75.5605) -> (57.0594, -73.3113) centre (53.1625, -71.0609) ccw
  circle A8 centre (53.7342, -72.0705) radius 1.1
  line L6 (-18.6227, 35.5765) -> (18.4839, 35.5734)
  line L7 (75.543, -25.8607) -> (75.543, -40.0977)
  arc A9 (74.9399, -42.3481) -> (75.543, -40.0977) centre (71.043, -40.0977) ccw
  line L8 (74.9399, -42.3481) -> (57.0594, -73.3113)
  line L9 (19.4614, 35.4658) -> (45.6471, 29.6358)
  circle A10 centre (18.5935, 32.0734) radius 1.1
  arc A11 (19.4614, 35.4658) -> (18.4839, 35.5734) centre (18.4835, 31.0734) ccw
  circle A12 centre (-51.125, 10.1813) radius 1.1
  line L10 (-52.6557, 13.373) -> (-21.1537, 34.7975)
  arc A13 (-18.6227, 35.5765) -> (-21.1537, 34.7975) centre (-18.6231, 31.0765) ccw
  circle A14 centre (-18.9309, 32.0765) radius 1.1
  arc A15 (-52.6557, 13.373) -> (-54.625, 9.652) centre (-50.125, 9.652) ccw
  circle A16 centre (-18.212, -50.5781) radius 1.1
  circle A17 centre (-51.125, -50.075) radius 1.1
  arc A18 (-16.9681, -55.0126) -> (-23.4871, -53.575) centre (-23.4871, -69.075) ccw
  line L11 (-50.125, -53.575) -> (-23.4871, -53.575)
  arc A19 (-54.625, -49.075) -> (-50.125, -53.575) centre (-50.125, -49.075) ccw
  line L12 (64, -16) -> (69, -16)
  line L13 (69, -16) -> (69, -26)
  line L14 (69, -26) -> (64, -26)
  line L15 (64, -26) -> (64, -16)
  constraint horizontal L12
  constraint vertical L13
  constraint horizontal L14
  constraint vertical L15
sketch "bottom_b" plane through (0, 0, 0) normal (0, 1, 0) x (1, 0, 0)
  line L0 (10.525, 23.075) -> (29.575, 23.075)
  line L1 (-27.575, -47.575) -> (-48.625, -47.575)
  circle A0 centre (-51.125, -50.075) radius 1.7
  line L2 (69.1916, -25.8629) -> (69.077, 25.397)
  line L3 (-29.575, 23.575) -> (-10.525, 23.575)
  line L4 (-29.575, 11.575) -> (-29.575, 23.575)
  circle A1 centre (-18.9309, 32.0765) radius 1.7
  line L5 (16.6792, -55.125) -> (-3.2391, -55.125)
  line L6 (-48.625, -47.575) -> (-48.625, 11.575)
  circle A2 centre (-18.212, -50.5781) radius 1.7
  circle A3 centre (-51.125, 10.1813) radius 1.7
  line L7 (-27.575, -35.575) -> (-27.575, -47.575)
  line L8 (50.4596, -69.0135) -> (34.8258, -59.9874)
  line L9 (29.575, 23.075) -> (29.575, 20.575)
  arc A4 (69.1916, -25.8629) -> (70.1916, -26.8607) centre (70.1916, -25.8607) ccw
  line L10 (47.625, 30.4938) -> (47.625, 20.575)
  circle A5 centre (71.1231, -41.9588) radius 1.7
  circle A6 centre (72.1849, -22.8607) radius 1.7
  line L11 (79.293, -40.0977) -> (79.293, -39.7668)
  circle A7 centre (18.5935, 32.0734) radius 1.7
  line L12 (69.6545, -38.7668) -> (76.593, -38.7668)
  line L13 (66.6131, -43.0348) -> (51.8256, -68.6475)
  line L14 (70.1916, -26.8607) -> (76.593, -26.8607)
  circle A8 centre (53.7342, -72.0705) radius 1.7
  circle A9 centre (72.1849, 20.1393) radius 1.7
  circle A10 centre (43.1794, 26.5995) radius 1.7
  line L15 (34.8258, -59.9874) -> (16.6792, -55.125)
  line L16 (29.575, 20.575) -> (47.625, 20.575)
  line L17 (-3.2391, -55.125) -> (-11.2391, -35.575)
  line L18 (-48.625, 11.575) -> (-29.575, 11.575)
  line L19 (-10.525, 23.575) -> (-10.525, 29.575)
  line L20 (10.525, 29.575) -> (10.525, 23.075)
  line L21 (-10.525, 29.575) -> (10.525, 29.575)
  line L22 (19.9069, 37.4668) -> (46.0926, 31.6368)
  arc A11 (19.9069, 37.4668) -> (18.484, 37.6234) centre (18.4835, 31.0734) ccw
  line L23 (-18.6225, 37.6265) -> (18.484, 37.6234)
  arc A12 (-18.6225, 37.6265) -> (-22.3066, 36.4926) centre (-18.6231, 31.0765) ccw
  line L24 (-53.8085, 15.0681) -> (-22.3066, 36.4926)
  arc A13 (-53.8085, 15.0681) -> (-56.675, 9.652) centre (-50.125, 9.652) ccw
  line L25 (-56.675, -49.075) -> (-56.675, 9.652)
  arc A14 (-56.675, -49.075) -> (-50.125, -55.625) centre (-50.125, -49.075) ccw
  line L26 (-50.125, -55.625) -> (-23.4871, -55.625)
  arc A15 (-17.8303, -56.8724) -> (-23.4871, -55.625) centre (-23.4871, -69.075) ccw
  line L27 (26.3037, -77.3319) -> (-17.8303, -56.8724)
  arc A16 (26.3037, -77.3319) -> (29.1477, -77.9388) centre (29.0585, -71.3894) ccw
  line L28 (53.2517, -77.6103) -> (29.1477, -77.9388)
  arc A17 (53.2517, -77.6103) -> (58.8346, -74.3365) centre (53.1625, -71.0609) ccw
  line L29 (76.7152, -43.3733) -> (58.8346, -74.3365)
  arc A18 (76.7152, -43.3733) -> (77.593, -40.0977) centre (71.043, -40.0977) ccw
  line L30 (46.0926, 31.6368) -> (46.8423, 31.4699)
  arc A19 (47.625, 30.4938) -> (46.8423, 31.4699) centre (46.625, 30.4938) ccw
  line L31 (77.593, -40.0977) -> (77.593, -39.7668)
  arc A20 (77.593, -39.7668) -> (76.593, -38.7668) centre (76.593, -39.7668) ccw
  line L32 (72.422, 25.7747) -> (70.3494, 26.3615)
  arc A21 (77.593, 19.3715) -> (72.422, 25.7747) centre (71.043, 19.3715) ccw
  line L33 (77.593, 19.3715) -> (77.593, -25.8607)
  arc A22 (70.3494, 26.3615) -> (69.077, 25.397) centre (70.077, 25.3993) ccw
  arc A23 (76.593, -26.8607) -> (77.593, -25.8607) centre (76.593, -25.8607) ccw
  line L34 (66.6131, -43.0348) -> (68.7885, -39.2668)
  arc A24 (69.6545, -38.7668) -> (68.7885, -39.2668) centre (69.6545, -39.7668) ccw
  line L35 (-27.575, -35.575) -> (-11.2391, -35.575)
  circle A25 centre (28.4977, -72.2317) radius 1.7
  arc A26 (50.4596, -69.0135) -> (51.8256, -68.6475) centre (50.9596, -68.1475) ccw
  dimension "d143" = 1
  dimension "d144" = 1
  dimension "d146" = 1
  dimension "d147" = 1
  dimension "d148" = 1
  dimension "d153" = 1
  constraint vertical L11
  constraint coincident L9.end L16.start
  constraint perpendicular L9 L16
  constraint parallel L22 L30
  constraint tangent L30 A19
  constraint tangent L10 A19
  constraint tangent A18 L31
  constraint vertical L31
  constraint tangent L12 A20
  constraint tangent L31 A20
  constraint tangent A17 L29
  constraint tangent L29 A18
  constraint tangent L28 A17
  constraint tangent A16 L28
  constraint tangent L27 A16
  constraint tangent A15 L27
  constraint tangent L26 A15
  constraint tangent A14 L26
  constraint tangent A13 L25
  constraint tangent A11 L23
  constraint tangent L24 A13
  constraint tangent A12 L24
  constraint tangent L22 A11
  constraint tangent L25 A14
  constraint tangent L23 A12
  constraint tangent A21 L33
  constraint tangent L2 A22
  constraint tangent L32 A22
  constraint tangent L33 A23
  constraint tangent L14 A23
  constraint parallel L13 L34
  constraint tangent L34 A24
  constraint tangent L12 A24
  constraint perpendicular L7 L35
  constraint tangent L8 A26
  constraint tangent L13 A26
  measures "d143" radius of A19
  measures "d144" radius of A20
  measures "d146" radius of A22
  measures "d147" radius of A23
  measures "d148" radius of A24
  measures "d153" radius of A26
sketch "bottom_c" plane through (0, 0, 0) normal (0, 1, 0) x (1, 0, 0)
  arc A0 (69.1916, -25.8629) -> (70.1916, -26.8607) centre (70.1916, -25.8607) ccw
  line L0 (79.293, -40.0977) -> (79.293, -39.7668)
  line L1 (69.6545, -38.7668) -> (78.293, -38.7668)
  line L2 (16.6792, -55.125) -> (-3.2391, -55.125)
  line L3 (46.462, 33.2962) -> (46.8423, 33.2115)
  circle A1 centre (72.1849, 20.1393) radius 1.7
  arc A2 (70.2865, 28.1461) -> (69.0691, 27.1678) centre (70.0691, 27.17) ccw
  line L4 (47.625, 32.2354) -> (47.625, 20.575)
  line L5 (-58.375, -49.075) -> (-58.375, 9.652)
  line L6 (79.293, 19.3715) -> (79.293, -25.8607)
  arc A3 (-18.5453, -58.4148) -> (-23.4871, -57.325) centre (-23.4871, -69.075) ccw
  arc A4 (47.625, 32.2354) -> (46.8423, 33.2115) centre (46.625, 32.2354) ccw
  line L7 (25.5887, -78.8743) -> (-18.5453, -58.4148)
  circle A5 centre (71.1231, -41.9588) radius 1.7
  line L8 (69.1916, -25.8629) -> (69.0729, 27.2561)
  arc A6 (-54.7645, 16.4738) -> (-58.375, 9.652) centre (-50.125, 9.652) ccw
  circle A7 centre (72.1849, -22.8607) radius 1.7
  line L9 (78.1873, -44.2234) -> (60.3068, -75.1866)
  arc A8 (79.293, 19.3715) -> (72.8359, 27.4243) centre (71.043, 19.3715) ccw
  line L10 (72.8359, 27.4243) -> (70.2865, 28.1461)
  circle A9 centre (43.1794, 26.5995) radius 1.7
  arc A10 (53.2749, -79.3102) -> (60.3068, -75.1866) centre (53.1625, -71.0609) ccw
  line L11 (20.2764, 39.1262) -> (46.462, 33.2962)
  line L12 (-48.625, -47.575) -> (-48.625, 11.575)
  circle A11 centre (-18.212, -50.5781) radius 1.7
  line L13 (-3.2391, -55.125) -> (-11.2391, -35.575)
  line L14 (-50.125, -57.325) -> (-23.4871, -57.325)
  arc A12 (-58.375, -49.075) -> (-50.125, -57.325) centre (-50.125, -49.075) ccw
  line L15 (-27.575, -47.575) -> (-48.625, -47.575)
  line L16 (-27.575, -35.575) -> (-27.575, -47.575)
  circle A13 centre (-51.125, -50.075) radius 1.7
  line L17 (-18.6224, 39.3265) -> (18.4842, 39.3234)
  line L18 (-29.575, 23.575) -> (-10.525, 23.575)
  line L19 (34.8258, -59.9874) -> (16.6792, -55.125)
  line L20 (29.575, 20.575) -> (47.625, 20.575)
  line L21 (53.2749, -79.3102) -> (29.1709, -79.6387)
  line L22 (29.575, 23.075) -> (29.575, 20.575)
  arc A14 (78.1873, -44.2234) -> (79.293, -40.0977) centre (71.043, -40.0977) ccw
  circle A15 centre (18.5935, 32.0734) radius 1.7
  line L23 (66.3631, -43.4678) -> (51.8256, -68.6475)
  arc A16 (20.2764, 39.1262) -> (18.4842, 39.3234) centre (18.4835, 31.0734) ccw
  line L24 (50.4596, -69.0135) -> (34.8258, -59.9874)
  arc A17 (-18.6224, 39.3265) -> (-23.2626, 37.8983) centre (-18.6231, 31.0765) ccw
  line L25 (-29.575, 11.575) -> (-29.575, 23.575)
  line L26 (-10.525, 23.575) -> (-10.525, 29.575)
  line L27 (-10.525, 29.575) -> (10.525, 29.575)
  line L28 (10.525, 29.575) -> (10.525, 23.075)
  line L29 (-48.625, 11.575) -> (-29.575, 11.575)
  circle A18 centre (53.7342, -72.0705) radius 1.7
  circle A19 centre (-51.125, 10.1813) radius 1.7
  circle A20 centre (-18.9309, 32.0765) radius 1.7
  line L30 (-54.7645, 16.4738) -> (-23.2626, 37.8983)
  line L31 (10.525, 23.075) -> (29.575, 23.075)
  line L32 (70.1916, -26.8607) -> (78.293, -26.8607)
  circle A21 centre (28.4977, -72.2317) radius 1.7
  arc A22 (78.293, -26.8607) -> (79.293, -25.8607) centre (78.293, -25.8607) ccw
  arc A23 (79.293, -39.7668) -> (78.293, -38.7668) centre (78.293, -39.7668) ccw
  arc A24 (25.5887, -78.8743) -> (29.1709, -79.6387) centre (29.0585, -71.3894) ccw
  line L33 (-27.575, -35.575) -> (-11.2391, -35.575)
  line L34 (66.3631, -43.4678) -> (68.7885, -39.2668)
  arc A25 (69.6545, -38.7668) -> (68.7885, -39.2668) centre (69.6545, -39.7668) ccw
  arc A26 (50.4596, -69.0135) -> (51.8256, -68.6475) centre (50.9596, -68.1475) ccw
  dimension "d149" = 1
  dimension "d150" = 1
  dimension "d151" = 1
  dimension "d152" = 1
  constraint coincident L8.end A2
  constraint tangent L0 A14
  constraint vertical L0
  constraint tangent L1 A23
  constraint tangent L0 A23
  constraint parallel L3 L11
  constraint tangent L3 A4
  constraint tangent L4 A4
  constraint coincident L20.start L22.end
  constraint perpendicular L20 L22
  constraint perpendicular L16 L33
  constraint parallel L23 L34
  constraint tangent L34 A25
  constraint tangent L1 A25
  constraint tangent L24 A26
  constraint tangent L23 A26
  measures "d149" radius of A23
  measures "d150" radius of A4
  measures "d151" radius of A25
  measures "d152" radius of A26
sketch "bottom_d" plane through (0, 0, 0) normal (0, 1, 0) x (1, 0, 0)
  line L0 (10.525, 23.075) -> (29.575, 23.075)
  circle A0 centre (72.1849, 20.1393) radius 1.7
  line L1 (-18.6223, 40.5765) -> (18.4843, 40.5734)
  line L2 (-50.125, -58.575) -> (-23.4871, -58.575)
  line L3 (-27.575, -47.575) -> (-48.625, -47.575)
  line L4 (-27.575, -35.575) -> (-27.575, -47.575)
  arc A1 (-59.625, -49.075) -> (-50.125, -58.575) centre (-50.125, -49.075) ccw
  line L5 (69.1916, -25.8629) -> (69.0702, 28.465)
  arc A2 (80.543, 19.3715) -> (73.1075, 28.6444) centre (71.043, 19.3715) ccw
  line L6 (-29.575, 23.575) -> (-10.525, 23.575)
  circle A3 centre (71.1231, -41.9588) radius 1.7
  line L7 (34.8258, -59.9874) -> (16.6792, -55.125)
  line L8 (70.1916, -26.8607) -> (79.543, -26.8607)
  line L9 (53.2919, -80.5601) -> (29.1879, -80.8885)
  arc A4 (80.5358, -39.7279) -> (79.5366, -38.7668) centre (79.5366, -39.7668) ccw
  line L10 (46.7337, 34.5163) -> (46.8423, 34.4921)
  line L11 (69.0702, 28.465) -> (69.0699, 28.4264)
  circle A5 centre (43.1794, 26.5995) radius 1.7
  arc A6 (79.543, -26.8607) -> (80.543, -25.8607) centre (79.543, -25.8607) ccw
  arc A7 (79.2698, -44.8485) -> (80.5358, -39.7279) centre (71.043, -40.0977) ccw
  line L12 (69.6545, -38.7668) -> (79.5366, -38.7668)
  arc A8 (47.625, 33.516) -> (46.8423, 34.4921) centre (46.625, 33.516) ccw
  arc A9 (69.1916, -25.8629) -> (70.1916, -26.8607) centre (70.1916, -25.8607) ccw
  line L13 (79.2698, -44.8485) -> (61.3893, -75.8117)
  line L14 (50.4596, -69.0135) -> (34.8258, -59.9874)
  arc A10 (53.2919, -80.5601) -> (61.3893, -75.8117) centre (53.1625, -71.0609) ccw
  circle A11 centre (53.7342, -72.0705) radius 1.7
  arc A12 (70.3273, 29.3852) -> (69.0699, 28.4264) centre (70.0698, 28.4189) ccw
  line L15 (73.1075, 28.6444) -> (70.2865, 29.3961)
  line L16 (80.543, -40.0977) -> (80.543, -39.4973)
  line L17 (70.2865, 29.3961) -> (70.3273, 29.3852)
  line L18 (66.3631, -43.4678) -> (51.8256, -68.6475)
  line L19 (-10.525, 23.575) -> (-10.525, 29.575)
  line L20 (-59.625, -49.075) -> (-59.625, 9.652)
  circle A13 centre (-18.9309, 32.0765) radius 1.7
  arc A14 (25.063, -80.0083) -> (29.1879, -80.8885) centre (29.0585, -71.3894) ccw
  circle A15 centre (18.5935, 32.0734) radius 1.7
  line L21 (-3.2391, -55.125) -> (-11.2391, -35.575)
  circle A16 centre (-18.212, -50.5781) radius 1.7
  arc A17 (-19.071, -59.5488) -> (-23.4871, -58.575) centre (-23.4871, -69.075) ccw
  line L22 (-48.625, -47.575) -> (-48.625, 11.575)
  line L23 (16.6792, -55.125) -> (-3.2391, -55.125)
  line L24 (25.063, -80.0083) -> (-19.071, -59.5488)
  line L25 (-10.525, 29.575) -> (10.525, 29.575)
  line L26 (69.0702, 28.465) -> (69.1309, 1.3011)
  line L27 (10.525, 29.575) -> (10.525, 23.075)
  line L28 (29.575, 20.575) -> (47.625, 20.575)
  line L29 (20.548, 40.3463) -> (46.7337, 34.5163)
  circle A18 centre (72.1849, -22.8607) radius 1.7
  line L30 (80.543, 19.3715) -> (80.543, -25.8607)
  arc A19 (-55.4675, 17.5074) -> (-59.625, 9.652) centre (-50.125, 9.652) ccw
  circle A20 centre (-51.125, 10.1813) radius 1.7
  line L31 (-29.575, 11.575) -> (-29.575, 23.575)
  line L32 (-48.625, 11.575) -> (-29.575, 11.575)
  arc A21 (-18.6223, 40.5765) -> (-23.9656, 38.9319) centre (-18.6231, 31.0765) ccw
  circle A22 centre (28.4977, -72.2317) radius 1.7
  line L33 (-55.4675, 17.5074) -> (-23.9656, 38.9319)
  line L34 (47.625, 20.575) -> (47.625, 33.516)
  circle A23 centre (-51.125, -50.075) radius 1.7
  line L35 (29.575, 23.075) -> (29.575, 20.575)
  arc A24 (20.548, 40.3463) -> (18.4843, 40.5734) centre (18.4835, 31.0734) ccw
  line L36 (-27.575, -35.575) -> (-11.2391, -35.575)
  line L37 (66.3631, -43.4678) -> (68.7885, -39.2668)
  arc A25 (50.4596, -69.0135) -> (51.8256, -68.6475) centre (50.9596, -68.1475) ccw
  arc A26 (69.6545, -38.7668) -> (68.7885, -39.2668) centre (69.6545, -39.7668) ccw
  dimension "d154" = 1
  dimension "d155" = 1
  dimension "d156" = 1
  dimension "d157" = 1
  constraint tangent A7 L16
  constraint perpendicular L12 L16
  constraint tangent A4 L12
  constraint tangent A4 A7
  constraint parallel L10 L29
  constraint tangent L10 A8
  constraint tangent A8 L34
  constraint coincident L28.start L35.end
  constraint perpendicular L28 L34
  constraint parallel L5 L26
  constraint parallel L15 L17
  constraint tangent L11 A12
  constraint tangent A12 L17
  constraint perpendicular L4 L36
  constraint parallel L18 L37
  constraint tangent L14 A25
  constraint tangent L18 A25
  constraint tangent L37 A26
  constraint tangent L12 A26
  constraint equal A25 A26
  measures "d154" radius of A4
  measures "d155" radius of A8
  measures "d156" radius of A12
  measures "d157" radius of A25